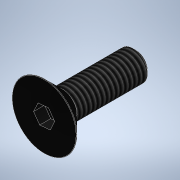
# Autodesk Inventor part: SCREW, FLAT HD, P, 12.9, M8X1.25X25MM
Saved by Autodesk Inventor 2022.4 (Build 264492000, 492)
## iProperties
Category: _
Manager: 100-05304
Shininess: 64.0
Length Units: 11269
Angle Units: 11279
Time Units: 11290
Mass Units: 11283
Length Display Precision: 3
Angle Display Precision: 2
Created: 2022-08-17
Part Number: SCREW, FLAT HD, P, 12.9, M8X1.25X25MM
Material: Default
Document SubType Name: Modeling
Designer: cdotson
Description: SCREW,FLAT HD,P,12.9,M8X1.25X025MM
Density: 1 g/cm^3
Appearance: Glossy - Black
Mfg Approved By: Bill.Nguyen
Mass: 1.62043 g
Surface Area: 11.1723 cm^2
Volume: 1.62043 cm^3
Engr Approved By: P
Checked By: 0003672579
User Status: Released
Density: 0.0
Volumn: 0.0
Area: 0.0
PropertySet Name: Model Information
Control State: 0
Master: False
Checked Out: False
CN_MASS: 0.0
PTC_WM_ITERATION: 2
PTC_WM_ORGANIZATION_ID: CLWC
PTC_WM_LIFECYCLE: CLWC_CAD_LC
FIRST_DESCRIPTION: M8X1.25X025MM
SECOND_DESCRIPTION: WV
THIRD_DESCRIPTION: _
CN_SERVICEABLE: _
ModelCat: Uncategorized
Author: -
Subject: FMPFHMA080125025
Keywords: DEFAULT
Revision Number: IR
Autodesk Inventor part; units mm, degrees
ref_plane "YZ Plane" through (0, 0, 0) normal (1, 0, 0) x (0, 1, 0)
ref_plane "XZ Plane" through (0, 0, 0) normal (0, 1, 0) x (-1, 0, 0)
ref_plane "XY Plane" through (0, 0, 0) normal (0, 0, 1) x (1, 0, 0)
sketch "Sketch1" plane through (0, 0, 0) normal (0, 0, 1) x (1, 0, 0)
  circle A0 centre (0, 0) radius 4
  dimension "Diameter" = 8
  constraints: 1 centre point
  measures "Diameter" diameter of A0
extrude "Extrusion1" add sketch "Sketch1" along normal blind 20.04
sketch "Sketch2" plane through (0, 0, 20.04) normal (0, 0, 1) x (1, 0, 0)
  circle A0 centre (0, 0) radius 4 projected
extrude "Extrusion2" add sketch "Sketch2" along normal blind 4.96 draft 45
sketch "Sketch3" plane through (0, 0, 25) normal (0, 0, 1) x (1, 0, 0)
  circle A0 centre (0, 0) radius 8.96 projected
  circle A1 centre (0, 0) radius 2.8868 construction
  line L0 (1.2084, 2.6217) -> (2.8746, 0.2644)
  line L1 (2.8746, 0.2644) -> (1.6662, -2.3573)
  line L2 (1.6662, -2.3573) -> (-1.2084, -2.6217)
  line L3 (-1.2084, -2.6217) -> (-2.8746, -0.2644)
  line L4 (-2.8746, -0.2644) -> (-1.6662, 2.3573)
  line L5 (-1.6662, 2.3573) -> (1.2084, 2.6217)
  dimension "Hex_Width" = 5
  constraints: 12 end point, 6 point on circle, 4 equal length, 1 centre point, 1 coincident
  measures "Hex_Width" distance between parallel lines of L0 L3
extrude "Extrusion3" cut sketch "Sketch3" against normal blind 3 contours L0 L1 L2 L3 L4 L5
thread "Thread1" size "M8x1.25" class "4g6g" standard "ANSI Metric M Profile" length 20.04
chamfer "Chamfer2" distance 0.8 angle 45 1 edges at (-4, 0, 0)
fillet "Fillet1" radius 0.1 1 edges at (-8.96, 0, 25)
equation "\"d10\" = Thread_Length"
equation "\"d13\" = Chamfer"
equation "\"Thread_Length\" = 20.04"
equation "\"Length\" = 25"
equation "\"Chamfer\" = 0.8"
body "Solid1"
